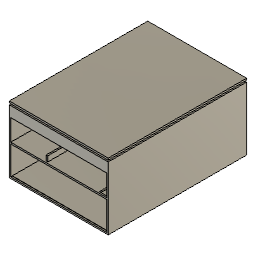
Water+level+sensor (Autodesk Fusion 360 design; units mm, degrees)
Autodesk Fusion 360 part; units mm, degrees
note: some values were not read from the file. Set by a fixed rule: which sketch regions a step uses.
sketch "Sketch1" plane through (0, 0, 0) normal (0, 0, 1) x (1, 0, 0)
  line L0 (0, 0) -> (54.2, 0)
  line L1 (54.2, 0) -> (54.2, 76.5)
  line L2 (54.2, 76.5) -> (0, 76.5)
  line L3 (0, 76.5) -> (0, 0)
  line L4 (-0.86, -0.86) -> (55.06, -0.86)
  line L5 (55.06, -0.86) -> (55.06, 77.36)
  line L6 (55.06, 77.36) -> (-0.86, 77.36)
  line L7 (-0.86, 77.36) -> (-0.86, -0.86)
  dimension "d1" = 54.2
  dimension "d2" = 76.5
  dimension "d5" = 0.86
  constraint horizontal L0
  constraint vertical L1
  constraint horizontal L2
  constraint vertical L3
  constraint coincident L0.start L3.end
  measures "d1" distance of L0.start L0.end
  measures "d2" distance of L0.start L2.end
extrude "Extrude2" add sketch "Sketch1" along normal blind 17 makes body 1
extrude "Extrude3" add sketch "Sketch1" along normal blind 1 contours L0 L1 L2 L3 bodies 1
sketch "Sketch2" plane through (0, 0, 17) normal (0, 0, 1) x (-1, 0, 0)
  line L0 (0, 0) -> (0, -76.5)
  line L1 (0, -76.5) -> (-54.2, -76.5)
  line L2 (-54.2, -76.5) -> (-54.2, 0)
  line L3 (-54.2, 0) -> (0, 0)
  line L4 (0.86, -77.36) -> (0.86, 0.86)
  line L5 (0.86, 0.86) -> (-55.06, 0.86)
  line L6 (-55.06, 0.86) -> (-55.06, -77.36)
  line L7 (-55.06, -77.36) -> (0.86, -77.36)
  line L8 (0.86, 0.86) -> (-55.06, 0.86)
  line L9 (-55.06, 0.86) -> (-55.06, -77.36)
  line L10 (-55.06, -77.36) -> (0.86, -77.36)
  line L11 (0.86, -77.36) -> (0.86, 0.86)
  line L12 (0, 0) -> (-54.2, 0)
  line L13 (-54.2, 0) -> (-54.2, -76.5)
  line L14 (-54.2, -76.5) -> (0, -76.5)
  line L15 (0, -76.5) -> (0, 0)
  line L16 (0, 0) -> (-5, 0)
  line L17 (-5, -23) -> (0, -23)
  line L18 (0, -23) -> (0, 0)
  line L19 (-5, -23) -> (0, -23)
  line L20 (0, -23) -> (0, -32)
  line L21 (0, -32) -> (-5, -32)
  line L22 (-5, -32) -> (-5, -23)
  line L23 (-54.2, 0) -> (-49.2, 0)
  line L24 (-49.2, 0) -> (-49.2, -20)
  line L25 (-49.2, -20) -> (-54.2, -20)
  line L26 (-54.2, -20) -> (-54.2, 0)
  dimension "d10" = -0.86
  dimension "d11" = 5
  dimension "d12" = 23
  dimension "d13" = 9
  dimension "d14" = 5
  dimension "d15" = 20
  constraint horizontal L8
  constraint vertical L9
  constraint horizontal L10
  constraint vertical L11
  constraint coincident L6.end L7.start
  constraint coincident L4.end L5.start
  constraint horizontal L16
  constraint horizontal L17
  constraint vertical L18
  constraint horizontal L19
  constraint vertical L20
  constraint horizontal L21
  constraint vertical L22
  constraint horizontal L23
  constraint vertical L24
  constraint horizontal L25
  constraint vertical L26
  measures "d11" distance of L0.start L16.end
  measures "d12" distance of L0.start L17.end
  measures "d13" distance of L17.start L21.end
  measures "d14" distance of L2.end L23.end
  measures "d15" distance of L2.end L25.end
extrude "Extrude4" add sketch "Sketch2" along normal blind 0.86 separate body contours L0 L1 L2 L3 L12 L13 L14 L15 L16 L17 L18 L19 L21 L22 L24 L25 makes body 2
extrude "Extrude5" add 1 faces at (-0.5733, 51, 17) along direction (0, 0, 1) blind 0.86 on bodies 1 bodies 1 2
sketch "Sketch3" plane through (0, -0.86, 0) normal (0, -1, 0) x (1, 0, 0)
  line L0 (-0.86, 0) -> (55.06, 0)
  line L1 (55.06, 0) -> (55.06, 17.86)
  line L2 (55.06, 17.86) -> (-0.86, 17.86)
  line L3 (-0.86, 17.86) -> (-0.86, 0)
  line L4 (-0.86, 0) -> (55.06, 0)
  line L5 (55.06, 0) -> (55.06, 17.86)
  line L6 (55.06, 17.86) -> (-0.86, 17.86)
  line L7 (-0.86, 17.86) -> (-0.86, 0)
  line L8 (0, 0.86) -> (54.2, 0.86)
  line L9 (54.2, 0.86) -> (54.2, 17)
  line L10 (54.2, 17) -> (0, 17)
  line L11 (0, 17) -> (0, 0.86)
  dimension "d20" = -0.86
  constraint horizontal L4
  constraint vertical L5
  constraint horizontal L6
  constraint vertical L7
  constraint coincident L1.end L2.start
  constraint coincident L0.start L3.end
extrude "Extrude6" cut sketch "Sketch3" against normal blind 0.86 contours L8 L9 L10 L11 bodies 1
sketch "Sketch12" plane through (0, 0, 17.86) normal (0, 0, 1) x (-1, 0, 0)
  line L0 (-49.2, 0) -> (-49.2, -20)
  line L1 (-49.2, -20) -> (-54.2, -20)
  line L2 (-54.2, -20) -> (-54.2, 0)
  line L3 (-54.2, 0) -> (-49.2, 0)
  line L4 (0.86, -77.36) -> (0.86, 0.86)
  line L5 (0.86, 0.86) -> (-55.06, 0.86)
  line L6 (-55.06, 0.86) -> (-55.06, -77.36)
  line L7 (-55.06, -77.36) -> (0.86, -77.36)
  line L8 (0, -23) -> (0, -32)
  line L9 (0, -32) -> (-5, -32)
  line L10 (-5, -32) -> (-5, -23)
  line L11 (-5, -23) -> (0, -23)
  line L12 (0.86, -77.36) -> (-55.06, -77.36)
  line L13 (-55.06, -77.36) -> (-55.06, 0.86)
  line L14 (0.86, 0.86) -> (0.86, -77.36)
  line L15 (-54.2, 0) -> (0, 0)
  line L16 (0, 0) -> (0, -76.5)
  line L17 (0, -76.5) -> (-54.2, -76.5)
  line L18 (-54.2, -76.5) -> (-54.2, 0)
  line L19 (0, -76.5) -> (-45.2, -76.5)
  line L20 (-45.2, -76.5) -> (-45.2, -59.5)
  line L21 (-45.2, -59.5) -> (0, -59.5)
  line L22 (0, -59.5) -> (0, -76.5)
  line L23 (-46.06, -76.5) -> (-46.06, -59.5)
  line L24 (-45.2, -58.64) -> (0, -58.64)
  line L25 (-45.2, -58.64) -> (-46.06, -58.64)
  line L26 (0, -58.64) -> (-48.5, -58.64)
  line L27 (-48.5, -58.64) -> (-48.5, -32.64)
  line L28 (0, -32.64) -> (0, -58.64)
  line L29 (0, -58.64) -> (-48.5, -58.64)
  line L30 (-48.5, -58.64) -> (-48.5, -31.94)
  line L31 (-48.5, -31.94) -> (0, -31.94)
  line L32 (0, -31.94) -> (0, -58.64)
  line L33 (-49.36, -58.64) -> (-49.36, -32.64)
  line L34 (-48.5, -31.08) -> (-5, -31.08)
  line L35 (-49.36, -32.64) -> (-49.36, -31.08)
  line L36 (-49.36, -31.08) -> (-48.5, -31.08)
  line L37 (-49.36, -58.64) -> (-49.36, -59.5)
  line L38 (-49.36, -59.5) -> (-46.06, -59.5)
  line L39 (-49.2, 0) -> (-20.1, 0)
  line L40 (-20.1, 0) -> (-20.1, -29.3)
  line L41 (-20.1, -29.3) -> (-49.2, -29.3)
  line L42 (-49.2, -29.3) -> (-49.2, 0)
  line L43 (-20.1, -30.16) -> (-49.2, -30.16)
  line L44 (-19.24, 0) -> (-19.24, -29.3)
  line L45 (-50.06, -29.3) -> (-50.06, -20)
  line L46 (-50.06, -29.3) -> (-50.06, -30.16)
  line L47 (-50.06, -30.16) -> (-49.2, -30.16)
  line L48 (-20.1, -30.16) -> (-19.24, -30.16)
  line L49 (-19.24, -30.16) -> (-19.24, -29.3)
  dimension "d40" = 0.86
  dimension "d41" = 45.2
  dimension "d42" = 17
  dimension "d43" = -0.86
  dimension "d44" = -0.86
  dimension "d45" = 48.5
  dimension "d47" = 48.5
  dimension "d52" = -0.86
  dimension "d53" = -0.86
  dimension "d54" = 29.1
  dimension "d55" = 29.3
  dimension "d56" = -0.86
  dimension "d57" = -0.86
  dimension "d58" = -0.86
  constraint horizontal L12
  constraint vertical L13
  constraint vertical L14
  constraint coincident L5.end L6.start
  constraint coincident L4.start L7.end
  constraint horizontal L19
  constraint vertical L20
  constraint horizontal L21
  constraint vertical L22
  constraint perpendicular L23 L25
  constraint horizontal L26
  constraint vertical L27
  constraint vertical L28
  constraint horizontal L29
  constraint vertical L30
  constraint horizontal L31
  constraint vertical L32
  constraint coincident L10 L34.end
  constraint perpendicular L34 L35
  constraint perpendicular L35 L36
  constraint perpendicular L21 L37
  constraint horizontal L39
  constraint vertical L40
  constraint horizontal L41
  constraint vertical L42
  constraint coincident L0.start L3.end
  constraint coincident L1 L45.end
  constraint perpendicular L43 L46
  constraint perpendicular L46 L47
  constraint perpendicular L44 L48
  constraint perpendicular L48 L49
  measures "d41" distance of L16.end L19.end
  measures "d42" distance of L16.end L21.end
  measures "d45" distance of L24.end L26.end
  measures "d47" distance of L24.end L26.end
  measures "d54" distance of L0.start L39.end
  measures "d55" distance of L0.start L41.end
extrude "Extrude10" add sketch "Sketch12" along normal blind 17.9 bodies 1
extrude "Extrude11" add sketch "Sketch12" along normal blind 3 contours L1 L15 L40 L41 L42 L43 L44 L45 L46 L47 L48 L49 | L10 L16 L17 L20 L21 L23 L24 L25 L26 L27 L29 L30 L31 L33 L34 L35 L36 L37 L38 bodies 1
sketch "Sketch13" plane through (0, -0.86, 0) normal (0, -1, 0) x (1, 0, 0)
  line L0 (54.2, 0.86) -> (0, 0.86)
  line L1 (0, 0.86) -> (0, 17)
  line L2 (0, 17) -> (54.2, 17)
  line L3 (54.2, 17) -> (54.2, 0.86)
  line L4 (-0.86, 0) -> (55.06, 0)
  line L5 (55.06, 0) -> (55.06, 35.76)
  line L6 (55.06, 35.76) -> (-0.86, 35.76)
  line L7 (-0.86, 35.76) -> (-0.86, 0)
  line L8 (54.2, 17) -> (54.2, 29.9)
  line L9 (54.2, 35.76) -> (0, 35.76)
  line L10 (0, 29.9) -> (0, 17)
  line L11 (54.2, 29.9) -> (0, 29.9)
  line L12 (0, 17) -> (54.2, 17)
  line L13 (0, 17.86) -> (54.2, 17.86)
  dimension "d65" = -0.86
  constraint vertical L8
  constraint horizontal L9
  constraint coincident L6 L9.start
  constraint coincident L1.end L2.start
  constraint perpendicular L9 L10
  constraint coincident L2.end L3.start
extrude "Extrude12" cut sketch "Sketch13" against normal blind 0.86 contours L8 L10 L11 L13 bodies 1
sketch "Sketch14" plane through (0, 0, 35.76) normal (0, 0, 1) x (-1, 0, 0)
  line L0 (-54.2, 0) -> (0, 0)
  line L1 (0, 0) -> (0, -76.5)
  line L2 (0, -76.5) -> (-54.2, -76.5)
  line L3 (-54.2, -76.5) -> (-54.2, 0)
  line L4 (0.86, 0.86) -> (-55.06, 0.86)
  line L5 (-55.06, 0.86) -> (-55.06, -77.36)
  line L6 (-55.06, -77.36) -> (0.86, -77.36)
  line L7 (0.86, -77.36) -> (0.86, 0.86)
  line L8 (0, -76.5) -> (-54.2, -76.5)
  line L9 (-54.2, -76.5) -> (-54.2, 0)
  line L10 (-54.2, 0) -> (0, 0)
  line L11 (0, 0) -> (0, -76.5)
  line L12 (-0.2, -76.3) -> (-54, -76.3)
  line L13 (-54, -76.3) -> (-54, -0.2)
  line L14 (-54, -0.2) -> (-0.2, -0.2)
  line L15 (-0.2, -0.2) -> (-0.2, -76.3)
  dimension "d68" = 0.2
  constraint horizontal L8
  constraint vertical L9
  constraint horizontal L10
  constraint vertical L11
  constraint coincident L0.start L3.end
  constraint coincident L1.end L2.start
extrude "Extrude13" add sketch "Sketch14" along normal blind 0.86 separate body contours L12 L13 L14 L15 makes body 3
sketch "Sketch15" plane through (0, 0, 36.62) normal (0, 0, 1) x (-1, 0, 0)
  line L0 (-0.2, -0.2) -> (-54, -0.2)
  line L1 (-54, -0.2) -> (-54, -76.3)
  line L2 (-54, -76.3) -> (-0.2, -76.3)
  line L3 (-0.2, -76.3) -> (-0.2, -0.2)
  line L4 (-55.06, -77.36) -> (0.86, -77.36)
  line L5 (0.86, -77.36) -> (0.86, 0.86)
  line L6 (0.86, 0.86) -> (-55.06, 0.86)
  line L7 (-55.06, 0.86) -> (-55.06, -77.36)
  dimension "d71" = 1.06
extrude "Extrude14" add sketch "Sketch15" along normal blind 1 contours L0 L1 L2 L3 | L4 L5 L6 L7 bodies 3
equation "d71 = 0.86 mm + 0.2 mm"
named bodies: "Arduino", "Lid"
